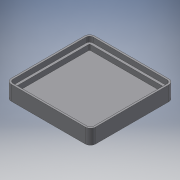
# Autodesk Inventor part: case_pantalla_3_inf
Saved by Autodesk Inventor 2019 (Build 230136000, 136)
## iProperties
Created: 2018-11-27
Part Number: case_pantalla_3_inf
Material: Genérico
Document SubType Name: Modeling
Designer: DIEGO 01
Density: 1 g/cm^3
Appearance: Por defecto
Author: DIEGO 01
Autodesk Inventor part; units mm, degrees
ref_plane "YZ Plane" through (0, 0, 0) normal (1, 0, 0) x (0, 1, 0)
ref_plane "XZ Plane" through (0, 0, 0) normal (0, 1, 0) x (-1, 0, 0)
ref_plane "XY Plane" through (0, 0, 0) normal (0, 0, 1) x (1, 0, 0)
sketch "Boceto1" plane through (0, 0, 0) normal (0, 1, 0) x (-1, 0, 0)
  line L0 (24.65, 24.4) -> (-24.65, 24.4)
  line L1 (-24.65, 24.4) -> (-24.65, -24.4)
  line L2 (-24.65, -24.4) -> (24.65, -24.4)
  line L3 (24.65, -24.4) -> (24.65, 24.4)
  line L4 (24.65, 24.4) -> (-24.65, -24.4) construction
  line L5 (-24.65, 24.4) -> (24.65, -24.4) construction
  point P0 (0, 0)
  dimension "d0" = 49.3
  dimension "d1" = 48.8
  constraints: 12 end point, 2 midpoint, 2 parallel, 1 horizontal, 1 perpendicular
  measures "d0" distance of L2.end L1.end
  measures "d1" distance of L1.end L0.end
extrude "Extrusión1" add sketch "Boceto1" against normal blind 8.4
fillet "Empalme1" radius 3 4 edges at (-24.65, -4.2, 24.4) (-24.65, -4.2, -24.4) (24.65, -4.2, -24.4) (24.65, -4.2, 24.4)
shell "Vaciado1" thickness 2.4 removed faces 1 at (7.2167, 0, -8.1333)
sketch "Boceto2" plane through (0, 0, 0) normal (0, 1, 0) x (1, 0, 0)
  arc A0 (22.25, 21.4) -> (21.65, 22) centre (21.65, 21.4) ccw projected
  line L0 (22.25, 21.4) -> (22.25, -21.4) projected
  arc A1 (21.65, -22) -> (22.25, -21.4) centre (21.65, -21.4) ccw projected
  line L1 (21.65, -22) -> (-21.65, -22) projected
  arc A2 (-22.25, -21.4) -> (-21.65, -22) centre (-21.65, -21.4) ccw projected
  line L2 (-22.25, -21.4) -> (-22.25, 21.4) projected
  arc A3 (-21.65, 22) -> (-22.25, 21.4) centre (-21.65, 21.4) ccw projected
  line L3 (-21.65, 22) -> (21.65, 22) projected
  arc A4 (21.65, -24.4) -> (24.65, -21.4) centre (21.65, -21.4) ccw projected
  line L4 (24.65, -21.4) -> (24.65, 21.4) projected
  arc A5 (24.65, 21.4) -> (21.65, 24.4) centre (21.65, 21.4) ccw projected
  line L5 (21.65, 24.4) -> (-21.65, 24.4) projected
  arc A6 (-21.65, 24.4) -> (-24.65, 21.4) centre (-21.65, 21.4) ccw projected
  line L6 (-24.65, 21.4) -> (-24.65, -21.4) projected
  arc A7 (-24.65, -21.4) -> (-21.65, -24.4) centre (-21.65, -21.4) ccw projected
  line L7 (-21.65, -24.4) -> (21.65, -24.4) projected
  line L8 (-23.65, 21.4) -> (-23.65, -21.4)
  arc A8 (-23.65, -21.4) -> (-21.65, -23.4) centre (-21.65, -21.4) ccw
  line L9 (-21.65, -23.4) -> (21.65, -23.4)
  arc A9 (21.65, -23.4) -> (23.65, -21.4) centre (21.65, -21.4) ccw
  line L10 (23.65, -21.4) -> (23.65, 21.4)
  arc A10 (23.65, 21.4) -> (21.65, 23.4) centre (21.65, 21.4) ccw
  line L11 (21.65, 23.4) -> (-21.65, 23.4)
  arc A11 (-21.65, 23.4) -> (-23.65, 21.4) centre (-21.65, 21.4) ccw
  point P0 (0, 0)
  dimension "d6" = 1.4
  constraints: 8 end point, 8 point on circle, 4 centre point, 7 other
  measures "d6" distance between parallel lines of L2 L8
extrude "Extrusión2" cut sketch "Boceto2" against normal blind 3 contours A11 L11 A10 L10 A9 L9 A8 L8
